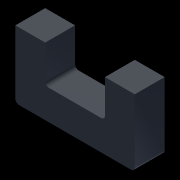
# Autodesk Inventor part: ferrite_core
Saved by Autodesk Inventor 2012 (Build 160160000, 160)
## iProperties
Created: 2012-10-11
Part Number: ferrite_core
Material: Default
Document SubType Name: Modeling
Designer: SONY
Density: 1 g/cm^3
Author: SONY
Autodesk Inventor part; units mm, degrees
ref_plane "YZ Plane" through (0, 0, 0) normal (1, 0, 0) x (0, 1, 0)
ref_plane "XZ Plane" through (0, 0, 0) normal (0, 1, 0) x (-1, 0, 0)
ref_plane "XY Plane" through (0, 0, 0) normal (0, 0, 1) x (1, 0, 0)
sketch "Sketch1" plane through (0, 0, 0) normal (0, 0, 1) x (1, 0, 0)
  line L0 (-21.2406, 0) -> (122.8406, 0) projected
  line L1 (0, -12.2191) -> (0, 68.7115) projected
  line L2 (3.175, 0) -> (98.425, 0)
  line L3 (101.6, 3.175) -> (101.6, 25.4)
  line L4 (73.025, 25.4) -> (28.575, 25.4)
  line L5 (0, 25.4) -> (0, 3.175)
  line L6 (0, 25.4) -> (25.4, 25.4)
  line L7 (25.4, 28.575) -> (25.4, 57.15)
  line L8 (25.4, 57.15) -> (0, 57.15)
  line L9 (0, 57.15) -> (0, 25.4)
  line L10 (76.2, 57.15) -> (101.6, 57.15)
  line L11 (101.6, 57.15) -> (101.6, 25.4)
  line L12 (101.6, 25.4) -> (76.2, 25.4)
  line L13 (76.2, 28.575) -> (76.2, 57.15)
  arc A0 (25.4, 28.575) -> (28.575, 25.4) centre (28.575, 28.575) ccw
  arc A1 (73.025, 25.4) -> (76.2, 28.575) centre (73.025, 28.575) ccw
  arc A2 (98.425, 0) -> (101.6, 3.175) centre (98.425, 3.175) ccw
  arc A3 (0, 3.175) -> (3.175, 0) centre (3.175, 3.175) ccw
  point P0 (0, 0)
  point P1 (101.6, 0)
  dimension "d0" = 101.6
  dimension "d1" = 25.4
  dimension "d2" = 25.4
  dimension "d3" = 57.15
  dimension "d4" = 25.4
  dimension "d5" = 57.15
  dimension "d6" = 3.175
  constraints: 24 end point, 8 point on circle, 8 point on line, 8 tangent, 6 parallel, 4 centre point, 3 equal radius, 3 horizontal, 3 perpendicular
  measures "d0" distance of point (0, 0) point (101.6, 0)
  measures "d1" distance of L5.start point (0, 0)
  measures "d2" distance between parallel lines of L7 L9
  measures "d3" distance between parallel lines of L0 L8
  measures "d4" distance between parallel lines of L11 L13
  measures "d5" distance between parallel lines of L2 L10
  measures "d6" radius of A0
extrude "Extrusion1" add sketch "Sketch1" along normal blind 25.4 contours A3 L1 L8 L7 A0 L4 A1 L13 L10 L11 L3 A2 L0
body "Solid1"
